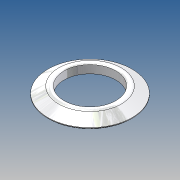
# Autodesk Inventor part: objektiv
Saved by Autodesk Inventor 2014 (Build 180170000, 170)
## iProperties
Created: 2011-11-30
Part Number: objektiv
Material: Generic
Document SubType Name: Modeling
Designer: slazh bliskovic
Density: 1 g/cm^3
Mass: 0.866835 g
Surface Area: 11.3272 cm^2
Volume: 0.866835 cm^3
Appearance: Aluminum - Polished
Author: slazh bliskovic
Autodesk Inventor part; units mm, degrees
ref_plane "YZ Plane" through (0, 0, 0) normal (1, 0, 0) x (0, 1, 0)
ref_plane "XZ Plane" through (0, 0, 0) normal (0, 1, 0) x (-1, 0, 0)
ref_plane "XY Plane" through (0, 0, 0) normal (0, 0, 1) x (1, 0, 0)
sketch "Sketch1" plane through (0, 0, 0) normal (0, 0, 1) x (1, 0, 0)
  circle A0 centre (24.0765, 0.0001) radius 15
  point P0 (0, 0)
  dimension "d0" = 30
  constraints: 1 centre point
  measures "d0" diameter of A0
extrude "Extrusion1" add sketch "Sketch1" along normal blind 3.5
chamfer "Chamfer1" distance 3 distance2 5 1 edges at (9.0765, 0.0001, 3.5) measured on face at (38.8822, -2.4061, 2.3333)
chamfer "Chamfer2" distance 0.25 angle 45 1 edges at (9.0765, 0.0001, 0)
sketch "Sketch2" plane through (24.0765, 0.0001, 3.5) normal (0, 0, 1) x (1, 0, 0)
  circle A0 centre (0, 0) radius 10 projected
  circle A1 centre (0, 0) radius 9.25
  point P0 (-24.0765, -0.0001)
  dimension "d9" = 18.5
  constraints: 1 centre point, 1 coincident
  measures "d9" diameter of A1
extrude "Extrusion2" cut sketch "Sketch2" against normal blind 0.65 contours A1
fillet "Fillet2" radius 2 2 edges at (14.8265, 0.0001, 3.5) (14.0765, 0.0001, 3.5)
sketch "Sketch3" plane through (24.0765, 0.0001, 2.85) normal (0, 0, 1) x (1, 0, 0)
  circle A0 centre (0, 0) radius 9.25 projected
  point P0 (-24.0765, -0.0001)
extrude "Extrusion3" cut sketch "Sketch3" against normal through all
body "Solid1"
